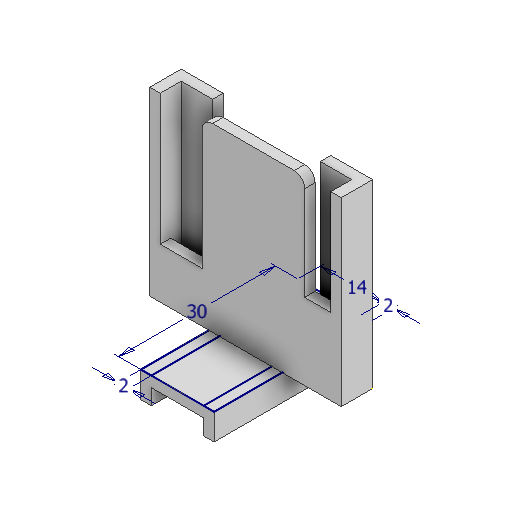
# Autodesk Inventor part: end effector
Saved by Autodesk Inventor 2025.3 (Build 293356030, 356C)
## iProperties
Created: 2025-10-16
Part Number: end effector
Material: 일반
Document SubType Name: Modeling
Designer: joseph
Density: 1 g/cm^3
Appearance: 기본값
Author: joseph
Autodesk Inventor part; units mm, degrees
ref_plane "YZ Plane" through (0, 0, 0) normal (1, 0, 0) x (0, 1, 0)
ref_plane "XZ Plane" through (0, 0, 0) normal (0, 1, 0) x (-1, 0, 0)
ref_plane "XY Plane" through (0, 0, 0) normal (0, 0, 1) x (1, 0, 0)
sketch "스케치1" plane through (0, 0, 0) normal (0, 1, 0) x (-1, 0, 0)
  line L0 (0, 0) -> (32.6, 0)
  line L1 (32.6, 0) -> (32.6, -2)
  line L2 (0, -2) -> (0, 0)
  line L3 (34.6, -4) -> (34.6, 2)
  line L4 (34.6, 2) -> (-2, 2)
  line L5 (-2, 2) -> (-2, -4)
  line L6 (26.6, -2) -> (26.6, -4)
  line L7 (6, -2) -> (6, -4)
  line L8 (32.6, -2) -> (26.6, -2)
  line L9 (6, -2) -> (0, -2)
  line L10 (-2, -4) -> (6, -4)
  line L11 (26.6, -4) -> (34.6, -4)
  dimension "d0" = 32.6
  dimension "d1" = 2
  dimension "d3" = 6
  dimension "d4" = 6
  constraints: 24 end point, 6 parallel, 6 perpendicular, 1 horizontal, 2 other
  measures "d0" distance of L1.end L2.start
  measures "d1" distance of L0.end L1.end
  measures "d3" distance from line of L2.start L7
  measures "d4" horizontal distance of L1.end L6.end
extrude "돌출1" add sketch "스케치1" along normal blind 32.6
sketch "스케치2" plane through (0, 0, 0) normal (0, -1, 0) x (1, 0, 0)
  line L0 (0, -2) -> (0, 0) projected
  line L1 (-6, -2) -> (0, -2) projected
  line L2 (-6, -4) -> (-6, -2) projected
  line L3 (2, -4) -> (-6, -4) projected
  line L4 (2, 2) -> (2, -4) projected
  line L5 (-34.6, 2) -> (2, 2) projected
  line L6 (-34.6, -4) -> (-34.6, 2) projected
  line L7 (-26.6, -4) -> (-34.6, -4) projected
  line L8 (-26.6, -2) -> (-26.6, -4) projected
  line L9 (-32.6, -2) -> (-26.6, -2) projected
  line L10 (-32.6, 0) -> (-32.6, -2) projected
  line L11 (0, 0) -> (-32.6, 0) projected
  line L12 (-6, -4) -> (-6, -2) projected
  line L13 (-6, -4) -> (-26.6, -4)
  constraints: 2 end point, 1 collinear
extrude "돌출2" add sketch "스케치2" along normal blind 2
sketch "스케치3" plane through (-34.6, 32.6, 2) normal (0, 0, 1) x (1, 0, 0)
  line L0 (2, -32.6) -> (2, 0) projected
  line L1 (2, 0) -> (10, 0)
  line L2 (10, 0) -> (10, -25)
  line L3 (10, -25) -> (2, -25)
  line L4 (2, -25) -> (2, 0)
  line L5 (0, 0) -> (36.6, 0) projected
  point P0 (34.6, -32.6)
  point P1 (2, -25)
  dimension "d9" = 8
  dimension "d10" = 25
  constraints: 8 end point, 2 parallel, 1 collinear, 1 horizontal, 1 perpendicular, 1 point on line
  measures "d9" distance of L2.end L3.end
  measures "d10" distance of L1.end L2.end
extrude "돌출3" cut sketch "스케치3" against normal blind 2
sketch "스케치4" plane through (0, -2, 0) normal (0, -1, 0) x (1, 0, 0)
  line L0 (-9.3, 15) -> (-23.3, 15)
  line L1 (-23.3, 15) -> (-23.3, -15)
  line L2 (-23.3, -15) -> (-9.3, -15)
  line L3 (-9.3, -15) -> (-9.3, 15)
  line L4 (-34.6, -4) -> (2, -4) projected
  line L5 (-9.3, 15) -> (-11.3, 15)
  line L6 (-11.3, 15) -> (-11.3, -15)
  line L7 (-11.3, -15) -> (-9.3, -15)
  line L8 (-9.3, -15) -> (-9.3, 15)
  line L9 (-23.3, -15) -> (-21.3, -15)
  line L10 (-21.3, -15) -> (-21.3, 15)
  line L11 (-21.3, 15) -> (-23.3, 15)
  line L12 (-23.3, 15) -> (-23.3, -15)
  line L13 (-21.3, 15) -> (-23.3, 15)
  line L14 (-23.3, 15) -> (-23.3, -15)
  line L15 (-23.3, -15) -> (-21.3, -15)
  line L16 (-21.3, -15) -> (-21.3, 15)
  point P0 (0, 0)
  point P1 (-16.3, -15)
  point P2 (-16.3, -4)
  point P3 (-9.3, 0)
  point P4 (-21.3, -4)
  point P5 (-23.3, -4)
  point P6 (-21.3, -4)
  dimension "d13" = 14
  dimension "d14" = 30
  dimension "d15" = 2
  dimension "d16" = 2
  constraints: 32 end point, 8 parallel, 4 horizontal, 4 perpendicular, 3 midpoint, 2 point on line, 1 horizontal alignment, 1 vertical alignment
  measures "d13" distance of L2.end L1.end
  measures "d14" distance of L1.end L0.end
  measures "d15" distance of L7.end L6.end
  measures "d16" distance of L11.end L10.end
extrude "돌출4" add sketch "스케치4" along normal blind 2
extrude "돌출5" add sketch "스케치4" along normal blind 5 contours L3 L4 L6 L0 | L3 L2 L6 L4 | L10 L4 L1 L0
extrude "돌출6" add sketch "스케치4" along normal blind 5 contours L10 L2 L1 L4
sketch "스케치5" plane through (-34.6, 32.6, 2) normal (0, 0, 1) x (1, 0, 0)
  line L0 (28.6, 0) -> (34.6, 0) projected
  line L1 (34.6, 0) -> (29.6, 0)
  line L2 (29.6, 0) -> (29.6, -20)
  line L3 (29.6, -20) -> (34.6, -20)
  line L4 (34.6, -20) -> (34.6, 0)
  point P0 (34.6, -32.6)
  dimension "d23" = 5
  dimension "d24" = 20
  constraints: 8 end point, 2 parallel, 1 horizontal, 1 perpendicular
  measures "d23" distance of L3.end L2.end
  measures "d24" distance of L2.end L1.end
extrude "돌출7" cut sketch "스케치5" against normal blind 2
fillet "모깎기1" radius 2 2 edges at (-5, 32.6, 1) (-24.6, 32.6, 1)
